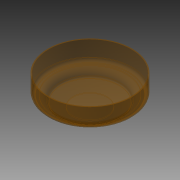
# Autodesk Inventor part: Case
Saved by Autodesk Inventor 2014 (Build 180170000, 170)
## iProperties
Created: 2014-10-26
Part Number: Case
Material: Polycarbonate, Smoke
Document SubType Name: Modeling
Designer: DV
Density: 1.2 g/cm^3
Appearance: Polycarbonate - Smoked
Mass: 0.0926949 g
Surface Area: 8.78293 cm^2
Volume: 0.0772458 cm^3
Author: DV
Autodesk Inventor part; units mm, degrees
ref_plane "YZ Plane" through (0, 0, 0) normal (1, 0, 0) x (0, 1, 0)
ref_plane "XZ Plane" through (0, 0, 0) normal (0, 1, 0) x (-1, 0, 0)
ref_plane "XY Plane" through (0, 0, 0) normal (0, 0, 1) x (1, 0, 0)
sketch "Sketch2" plane through (0, 0, 0) normal (0, 0, 1) x (1, 0, 0)
  line L0 (-8, -119.2353) -> (-8, -116.9353)
  line L1 (-6, -122.7333) -> (6, -122.7333) construction
  line L2 (0, -124.2363) -> (0, -116.6139)
  line L3 (-7.758, -121.6353) -> (-6.858, -121.6353) projected
  line L4 (1.9209, -117.9353) -> (-6, -117.9353) construction
  line L5 (3.2643, -119.9353) -> (-5.8702, -119.9353) construction
  line L6 (-8.254, -121.1393) -> (-8.254, -118.0642)
  line L7 (0, -123.7431) -> (-3.3921, -123.7431)
  arc A0 (-8.254, -121.1393) -> (-7.758, -121.6353) centre (-7.758, -121.1393) ccw
  line L8 (-7.758, -121.6353) -> (-7.2484, -121.6353)
  line L9 (-3.3921, -123.7431) -> (-5.8158, -122.9555)
  arc A1 (-6, -122.7333) -> (-5.8158, -122.9555) centre (-5.7324, -122.6988) ccw
  arc A2 (-6, -122.7333) -> (-7.2484, -121.6353) centre (-7.2484, -122.894) ccw
  line L10 (-8.4318, -118.1834) -> (-8.4318, -121.1393)
  arc A3 (-8.4318, -121.1393) -> (-7.758, -121.8131) centre (-7.758, -121.1393) ccw
  line L11 (-7.758, -121.8131) -> (-7.2484, -121.8131)
  arc A4 (-6.1763, -122.756) -> (-7.2484, -121.8131) centre (-7.2484, -122.894) ccw
  arc A5 (-6.1763, -122.756) -> (-5.8707, -123.1246) centre (-5.7324, -122.6988) ccw
  line L12 (-5.8707, -123.1246) -> (-3.4203, -123.9209)
  line L13 (-3.4203, -123.9209) -> (0, -123.9209)
  line L14 (0, -123.9209) -> (0, -123.7431)
  arc A6 (-8.254, -118.0642) -> (-8.4318, -118.1834) centre (-8.3829, -118.0642) ccw
  point P0 (0, 0)
  point P1 (-8.3829, -117.9353)
  dimension "d8" = 2
  dimension "d9" = 0.254
  dimension "d10" = 0.1778
  constraints: 24 end point, 15 point on circle, 7 centre point, 6 tangent, 3 perpendicular, 2 parallel, 2 point on line, 1 coincident, 1 collinear, 1 vertical, 6 other
  measures "d8" distance between parallel lines of L4 L5
  measures "d9" distance between parallel lines of L6 L0
  measures "d10" distance between parallel lines of L10 L6
revolve "Revolution1" add sketch "Sketch2" angle 360 about axis through (0, -124.2363, 0) along (0, 1, 0)
body "Solid1"
